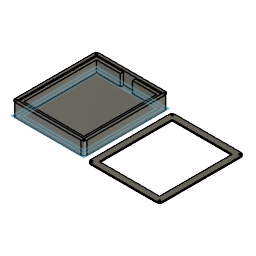
stopuhr gehäuse (Autodesk Fusion 360 design; units mm, degrees)
description: KiCad electronic assembly
part number: stopuhr 1
part number: PinSocket_1x01_P2.54mm_Vertical
part number: D_DO-41_SOD81_P10.16mm_Horizontal
part number: R_Axial_DIN0207_L6.3mm_D2.5mm_P7.62mm_Horizontal
part number: HDSP-7401
part number: CP_Radial_D5.0mm_P2.00mm
part number: DIP-8_W7.62mm
part number: stopuhr_PCB
Autodesk Fusion 360 part; units mm, degrees
sketch "Skizze1" plane through (0, 0, 0) normal (0, 0, 1) x (1, 0, 0)
  line L0 (20, 225) -> (129.29, 225)
  line L1 (129.29, 225) -> (129.29, 94.96)
  line L2 (129.29, 94.96) -> (20, 94.96)
  line L3 (20, 94.96) -> (20, 225)
  line L4 (15, 230) -> (134.29, 230)
  line L5 (134.29, 230) -> (134.29, 89.96)
  line L6 (134.29, 89.96) -> (15, 89.96)
  line L7 (15, 89.96) -> (15, 230)
  line L8 (25, 220) -> (124.29, 220)
  line L9 (124.29, 220) -> (124.29, 99.96)
  line L10 (124.29, 99.96) -> (25, 99.96)
  line L11 (25, 99.96) -> (25, 220)
  dimension "d1" = 109.29
  dimension "d2" = 130.04
  dimension "d3" = 119.29
  dimension "d4" = 140.04
  dimension "d5" = 5
  dimension "d6" = 5
  dimension "d7" = 99.29
  dimension "d8" = 120.04
  dimension "d9" = 5
  dimension "d10" = 5
  constraint horizontal L0
  constraint vertical L1
  constraint horizontal L2
  constraint vertical L3
  constraint horizontal L4
  constraint vertical L5
  constraint horizontal L6
  constraint vertical L7
  constraint horizontal L8
  constraint vertical L9
  constraint horizontal L10
  constraint vertical L11
  measures "d1" distance of L0.start L0.end
  measures "d2" distance of L0.start L2.end
  measures "d3" distance of L4.start L4.end
  measures "d4" distance of L4.start L6.end
  measures "d5" distance of L3 L7
  measures "d6" distance of L0 L4
  measures "d7" distance of L8.start L8.end
  measures "d8" distance of L8.start L10.end
  measures "d9" distance of L0 L8
  measures "d10" distance of L3 L11
extrude "Extrusion1" add sketch "Skizze1" along normal blind 1 contours L8 L9 L10 L11 makes body 1
extrude "Extrusion2" add sketch "Skizze1" along normal blind 20 contours L0 L1 L2 L3 bodies 1
extrude "Extrusion3" add sketch "Skizze1" along normal blind 22 contours L4 L5 L6 L7 bodies 1
sketch "Skizze2" plane through (0, 0, 20) normal (0, 0, 1) x (-1, 0, 0)
  line L0 (-124.29, -99.96) -> (-25, -99.96)
  line L1 (-25, -99.96) -> (-25, -220)
  line L2 (-25, -220) -> (-124.29, -220)
  line L3 (-124.29, -220) -> (-124.29, -99.96)
  line L4 (-20, -94.96) -> (-129.29, -94.96)
  line L5 (-129.29, -94.96) -> (-129.29, -225)
  line L6 (-129.29, -225) -> (-20, -225)
  line L7 (-20, -225) -> (-20, -94.96)
  line L8 (-64.5, -225) -> (-84.5, -225)
  line L9 (-84.5, -225) -> (-84.5, -220)
  line L10 (-84.5, -220) -> (-64.5, -220)
  line L11 (-64.5, -220) -> (-64.5, -225)
  line L12 (-20, -94.96) -> (-20, -225)
  dimension "d17" = 20
  dimension "d18" = 44.5
  constraint horizontal L8
  constraint vertical L9
  constraint horizontal L10
  constraint vertical L11
  constraint coincident L6 L8.start
  measures "d17" distance of L8.start L8.end
  measures "d18" distance of L11 L12
extrude "Extrusion4" cut sketch "Skizze2" against normal blind 19 contours L2 L6 L8 L9 L10 L11 bodies 1
sketch "Skizze3" plane through (0, 0, 22) normal (0, 0, 1) x (-1, 0, 0)
  line L0 (-129.29, -94.96) -> (-20, -94.96)
  line L1 (-20, -94.96) -> (-20, -225)
  line L2 (-20, -225) -> (-129.29, -225)
  line L3 (-129.29, -225) -> (-129.29, -94.96)
  line L4 (-15, -89.96) -> (-134.29, -89.96)
  line L5 (-134.29, -89.96) -> (-134.29, -230)
  line L6 (-134.29, -230) -> (-15, -230)
  line L7 (-15, -230) -> (-15, -89.96)
  circle A0 centre (-18.5, -226.5) radius 1.7
  line L8 (-20, -94.96) -> (-20, -225)
  circle A1 centre (-130.79, -226.5) radius 2
  line L9 (-129.29, -225) -> (-129.29, -94.96)
  line L10 (-20, -225) -> (-129.29, -225)
  circle A2 centre (-130.79, -93.46) radius 1.7
  line L11 (-129.29, -94.96) -> (-20, -94.96)
  circle A3 centre (-18.5, -93.46) radius 1.7
  dimension "d21" = 3.4
  dimension "d22" = 1.5
  dimension "d23" = 1.5
  dimension "d24" = 4
  dimension "d25" = 1.5
  dimension "d26" = 1.5
  dimension "d27" = 3.4
  dimension "d28" = 1.5
  dimension "d29" = 1.5
  dimension "d30" = 3.4
  dimension "d31" = 1.5
  dimension "d32" = 1.5
  measures "d21" diameter of A0
  measures "d22" vertical distance of L1.end A0.centre
  measures "d23" distance of A0.centre L8
  measures "d24" diameter of A1
  measures "d25" distance of A1.centre L9
  measures "d26" distance of A1.centre L10
  measures "d27" diameter of A2
  measures "d28" distance of A2.centre L11
  measures "d29" distance of L9 A2.centre
  measures "d30" diameter of A3
  measures "d31" distance of L11 A3.centre
  measures "d32" distance of L8 A3.centre
fillet "Abrundung1" radius 5 3 edges at (15, 230, 11) (134.29, 230, 11) (15, 89.96, 11) on bodies 1
fillet "Abrundung2" radius 5 1 edges at (134.29, 89.96, 11) on bodies 1
extrude "Extrusion5" cut sketch "Skizze3" against normal blind 19 contours A0 | A1 | A2 | A3 bodies 1
sketch "Skizze4" plane through (0, 0, 0) normal (0, 0, 1) x (1, 0, 0)
  line L0 (180, 225) -> (289.29, 225)
  line L1 (294.29, 220) -> (294.29, 89.96)
  line L2 (289.29, 84.96) -> (180, 84.96)
  line L3 (175, 89.96) -> (175, 220)
  line L4 (185, 215) -> (284.29, 215)
  line L5 (284.29, 215) -> (284.29, 94.96)
  line L6 (284.29, 94.96) -> (185, 94.96)
  line L7 (185, 94.96) -> (185, 215)
  circle A0 centre (290.79, 221.5) radius 1.7
  circle A1 centre (178.5, 221.5) radius 1.7
  circle A2 centre (178.5, 88.46) radius 1.7
  circle A3 centre (290.79, 88.46) radius 1.7
  arc A4 (289.29, 84.96) -> (294.29, 89.96) centre (289.29, 89.96) ccw
  arc A5 (175, 89.96) -> (180, 84.96) centre (180, 89.96) ccw
  arc A6 (294.29, 220) -> (289.29, 225) centre (289.29, 220) ccw
  arc A7 (180, 225) -> (175, 220) centre (180, 220) ccw
  point P0 (175, 225)
  point P1 (294.29, 225)
  point P2 (175, 84.96)
  dimension "d44" = 119.29
  dimension "d45" = 140.04
  dimension "d46" = 99.29
  dimension "d47" = 120.04
  dimension "d48" = 10
  dimension "d49" = 10
  dimension "d50" = 3.4
  dimension "d51" = 6.5
  dimension "d52" = 6.5
  dimension "d53" = 3.4
  dimension "d54" = 6.5
  dimension "d55" = 6.5
  dimension "d56" = 3.4
  dimension "d57" = 6.5
  dimension "d58" = 6.5
  dimension "d59" = 3.4
  dimension "d60" = 6.5
  dimension "d61" = 6.5
  dimension "d62" = 5
  dimension "d63" = 5
  dimension "d64" = 5
  dimension "d65" = 5
  constraint horizontal L0
  constraint vertical L1
  constraint horizontal L2
  constraint vertical L3
  constraint horizontal L4
  constraint vertical L5
  constraint horizontal L6
  constraint vertical L7
  constraint tangent L1 A4
  constraint tangent L2 A4
  constraint coincident P2 L2
  constraint coincident P2 L3
  constraint tangent L2 A5
  constraint tangent L3 A5
  constraint coincident P1 L0
  constraint coincident P1 L1
  constraint tangent L0 A6
  constraint tangent L1 A6
  constraint coincident P0 L0
  constraint coincident P0 L3
  constraint tangent L0 A7
  constraint tangent L3 A7
  measures "d44" distance of P0 P1
  measures "d45" distance of P0 P2
  measures "d46" distance of L4.start L4.end
  measures "d47" distance of L4.start L6.end
  measures "d48" distance of L0 L4
  measures "d49" distance of L3 L7
  measures "d50" diameter of A0
  measures "d51" distance of L4 A0.centre
  measures "d52" distance of L5 A0.centre
  measures "d53" diameter of A1
  measures "d54" distance of L4 A1.centre
  measures "d55" distance of L7 A1.centre
  measures "d56" diameter of A2
  measures "d57" distance of L6 A2.centre
  measures "d58" distance of L7 A2.centre
  measures "d59" diameter of A3
  measures "d60" distance of L5 A3.centre
  measures "d61" distance of L6 A3.centre
  measures "d62" radius of A4
  measures "d63" radius of A5
  measures "d64" radius of A6
  measures "d65" radius of A7
extrude "Extrusion6" add sketch "Skizze4" along normal blind 2 separate body makes body 2
move_body "Verschieben1" bodies 2 to x (1, 0, 0) y (0, 1, 0) z (0, 0, 1) at (-30, 0, 0)
component "R_Axial_DIN0207_L6.3mm_D2.5mm_P7.62mm_Horizontal" placed x (0, 1, 0) y (-1, 0, 0) z (0, 0, 1) at (85.01, -80.69, 1.595)
component "CP_Radial_D5.0mm_P2.00mm" placed x (1, 0, 0) y (0, 1, 0) z (0, 0, 1) at (76.42, -104.39, 1.595)
component "R_Axial_DIN0207_L6.3mm_D2.5mm_P7.62mm_Horizontal" placed x (-1, 0, 0) y (0, -1, 0) z (0, 0, 1) at (117.99, -130.58, 1.595)
component "R_Axial_DIN0207_L6.3mm_D2.5mm_P7.62mm_Horizontal" placed x (1, 0, 0) y (0, 1, 0) z (0, 0, 1) at (88.22, -55.43, 1.595)
component "R_Axial_DIN0207_L6.3mm_D2.5mm_P7.62mm_Horizontal" placed x (1, 0, 0) y (0, 1, 0) z (0, 0, 1) at (81.99, -106.71, 1.595)
component "PinSocket_1x01_P2.54mm_Vertical" placed x (1, 0, 0) y (0, 1, 0) z (0, 0, 1) at (118.605, -22.175, 1.595)
component "R_Axial_DIN0207_L6.3mm_D2.5mm_P7.62mm_Horizontal" placed x (1, 0, 0) y (0, 1, 0) z (0, 0, 1) at (153.3825, -46.8425, 1.595)
component "R_Axial_DIN0207_L6.3mm_D2.5mm_P7.62mm_Horizontal" placed x (0, 1, 0) y (-1, 0, 0) z (0, 0, 1) at (88.06, -80.77, 1.595)
component "R_Axial_DIN0207_L6.3mm_D2.5mm_P7.62mm_Horizontal" placed x (-1, 0, 0) y (0, -1, 0) z (0, 0, 1) at (141.62, -43.7, 1.595)
component "R_Axial_DIN0207_L6.3mm_D2.5mm_P7.62mm_Horizontal" placed x (0, 1, 0) y (-1, 0, 0) z (0, 0, 1) at (109.44, -71.18, 1.595)
component "CP_Radial_D5.0mm_P2.00mm" placed x (0, 1, 0) y (-1, 0, 0) z (0, 0, 1) at (105.38, -138.0151, 1.595)
component "CP_Radial_D5.0mm_P2.00mm" placed x (0, -1, 0) y (1, 0, 0) z (0, 0, 1) at (141.3, -76.71, 1.595)
component "DIP-8_W7.62mm" placed x (1, 0, 0) y (0, 1, 0) z (0, 0, 1) at (82.275, -90.82, 1.595)
component "R_Axial_DIN0207_L6.3mm_D2.5mm_P7.62mm_Horizontal" placed x (0, 1, 0) y (-1, 0, 0) z (0, 0, 1) at (125.49, -72.12, 1.595)
component "CP_Radial_D5.0mm_P2.00mm" placed x (1, 0, 0) y (0, 1, 0) z (0, 0, 1) at (114.7499, -32.595, 1.595)
component "R_Axial_DIN0207_L6.3mm_D2.5mm_P7.62mm_Horizontal" placed x (1, 0, 0) y (0, 1, 0) z (0, 0, 1) at (153.3825, -49.9025, 1.595)
component "R_Axial_DIN0207_L6.3mm_D2.5mm_P7.62mm_Horizontal" placed x (0, 1, 0) y (-1, 0, 0) z (0, 0, 1) at (106.42, -71.26, 1.595)
component "R_Axial_DIN0207_L6.3mm_D2.5mm_P7.62mm_Horizontal" placed x (-1, 0, 0) y (0, -1, 0) z (0, 0, 1) at (109.83, -124.51, 1.595)
component "R_Axial_DIN0207_L6.3mm_D2.5mm_P7.62mm_Horizontal" placed x (-1, 0, 0) y (0, -1, 0) z (0, 0, 1) at (76.46, -48.4, 1.595)
component "R_Axial_DIN0207_L6.3mm_D2.5mm_P7.62mm_Horizontal" placed x (1, 0, 0) y (0, 1, 0) z (0, 0, 1) at (88.3, -52.35, 1.595)
component "CP_Radial_D5.0mm_P2.00mm" placed x (0, 1, 0) y (-1, 0, 0) z (0, 0, 1) at (134.24, -99.41, 1.595)
component "R_Axial_DIN0207_L6.3mm_D2.5mm_P7.62mm_Horizontal" placed x (1, 0, 0) y (0, 1, 0) z (0, 0, 1) at (88.22, -43.22, 1.595)
component "R_Axial_DIN0207_L6.3mm_D2.5mm_P7.62mm_Horizontal" placed x (-1, 0, 0) y (0, -1, 0) z (0, 0, 1) at (141.5225, -55.9825, 1.595)
component "R_Axial_DIN0207_L6.3mm_D2.5mm_P7.62mm_Horizontal" placed x (-1, 0, 0) y (0, -1, 0) z (0, 0, 1) at (76.46, -51.5, 1.595)
component "R_Axial_DIN0207_L6.3mm_D2.5mm_P7.62mm_Horizontal" placed x (1, 0, 0) y (0, 1, 0) z (0, 0, 1) at (88.12, -46.3, 1.595)
component "R_Axial_DIN0207_L6.3mm_D2.5mm_P7.62mm_Horizontal" placed x (0, 1, 0) y (-1, 0, 0) z (0, 0, 1) at (137.88, -72.11, 1.595)
component "R_Axial_DIN0207_L6.3mm_D2.5mm_P7.62mm_Horizontal" placed x (0, 1, 0) y (-1, 0, 0) z (0, 0, 1) at (134.8, -72.09, 1.595)
component "R_Axial_DIN0207_L6.3mm_D2.5mm_P7.62mm_Horizontal" placed x (1, 0, 0) y (0, 1, 0) z (0, 0, 1) at (88.25, -49.3, 1.595)
component "R_Axial_DIN0207_L6.3mm_D2.5mm_P7.62mm_Horizontal" placed x (0, 1, 0) y (-1, 0, 0) z (0, 0, 1) at (128.57, -72.19, 1.595)
component "PinSocket_1x01_P2.54mm_Vertical" placed x (1, 0, 0) y (0, 1, 0) z (0, 0, 1) at (112.315, -22.175, 1.595)
component "R_Axial_DIN0207_L6.3mm_D2.5mm_P7.62mm_Horizontal" placed x (1, 0, 0) y (0, 1, 0) z (0, 0, 1) at (82.52, -102.66, 1.595)
component "HDSP-7401" placed x (1, 0, 0) y (0, 1, 0) z (0, 0, 1) at (116.9225, -44.5025, 1.595)
component "R_Axial_DIN0207_L6.3mm_D2.5mm_P7.62mm_Horizontal" placed x (-1, 0, 0) y (0, -1, 0) z (0, 0, 1) at (141.5325, -52.9325, 1.595)
component "HDSP-7401" placed x (1, 0, 0) y (0, 1, 0) z (0, 0, 1) at (108.4, -44.52, 1.595)
component "HDSP-7401" placed x (1, 0, 0) y (0, 1, 0) z (0, 0, 1) at (125.3, -44.48, 1.595)
component "R_Axial_DIN0207_L6.3mm_D2.5mm_P7.62mm_Horizontal" placed x (0, 1, 0) y (-1, 0, 0) z (0, 0, 1) at (131.7, -72.14, 1.595)
component "D_DO-41_SOD81_P10.16mm_Horizontal" placed x (0, 1, 0) y (-1, 0, 0) z (0, 0, 1) at (96.755, -100.16, 1.595)
component "R_Axial_DIN0207_L6.3mm_D2.5mm_P7.62mm_Horizontal" placed x (0, -1, 0) y (1, 0, 0) z (0, 0, 1) at (132.23, -83.97, 1.595)
component "CP_Radial_D5.0mm_P2.00mm" placed x (0, -1, 0) y (1, 0, 0) z (0, 0, 1) at (113.37, -76.09, 1.595)
component "R_Axial_DIN0207_L6.3mm_D2.5mm_P7.62mm_Horizontal" placed x (-1, 0, 0) y (0, -1, 0) z (0, 0, 1) at (141.46, -49.89, 1.595)
component "R_Axial_DIN0207_L6.3mm_D2.5mm_P7.62mm_Horizontal" placed x (0, -1, 0) y (1, 0, 0) z (0, 0, 1) at (135.32, -84.02, 1.595)
component "R_Axial_DIN0207_L6.3mm_D2.5mm_P7.62mm_Horizontal" placed x (-1, 0, 0) y (0, -1, 0) z (0, 0, 1) at (141.57, -46.85, 1.595)
component "R_Axial_DIN0207_L6.3mm_D2.5mm_P7.62mm_Horizontal" placed x (0, 1, 0) y (-1, 0, 0) z (0, 0, 1) at (96.89, -71.22, 1.595)
component "HDSP-7401" placed x (1, 0, 0) y (0, 1, 0) z (0, 0, 1) at (99.9925, -44.4625, 1.595)
component "CP_Radial_D5.0mm_P2.00mm" placed x (0, 1, 0) y (-1, 0, 0) z (0, 0, 1) at (156.49, -57.1751, 1.595)
component "R_Axial_DIN0207_L6.3mm_D2.5mm_P7.62mm_Horizontal" placed x (0, 1, 0) y (-1, 0, 0) z (0, 0, 1) at (100.07, -71.26, 1.595)
component "CP_Radial_D5.0mm_P2.00mm" placed x (0, -1, 0) y (1, 0, 0) z (0, 0, 1) at (76.725, -90.92, 1.595)
component "CP_Radial_D5.0mm_P2.00mm" placed x (0, 1, 0) y (-1, 0, 0) z (0, 0, 1) at (75.82, -98.52, 1.595)
component "R_Axial_DIN0207_L6.3mm_D2.5mm_P7.62mm_Horizontal" placed x (0, 1, 0) y (-1, 0, 0) z (0, 0, 1) at (103.27, -71.2, 1.595)
component "CP_Radial_D5.0mm_P2.00mm" placed x (-1, 0, 0) y (0, -1, 0) z (0, 0, 1) at (83.3, -59.8, 1.595)
component "stopuhr_PCB" placed x (1, 0, 0) y (0, 1, 0) z (0, 0, 1) at (0, 0, 0)
